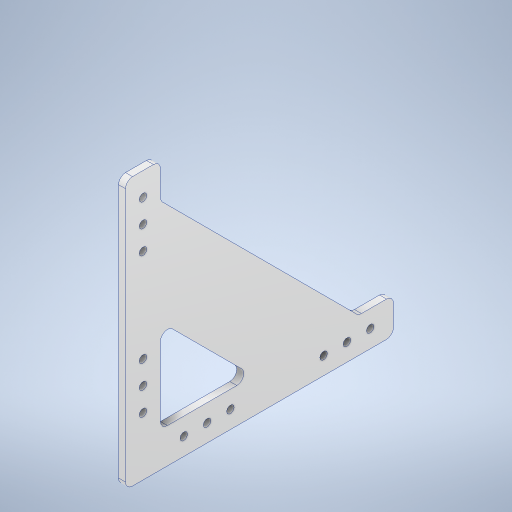
# Autodesk Inventor part: 射出_固定2
Saved by Autodesk Inventor 2023 (Build 270158000, 158)
## iProperties
Created: 2022-04-20
Part Number: 射出_固定2
Material: アルミニウム 6061
Document SubType Name: Modeling
Designer: yuta
Density: 2.7 g/cm^3
Appearance: アルミニウム - フラット
Author: yuta
Autodesk Inventor part; units mm, degrees
ref_plane "YZ Plane" through (0, 0, 0) normal (1, 0, 0) x (0, 1, 0)
ref_plane "XZ Plane" through (0, 0, 0) normal (0, 1, 0) x (-1, 0, 0)
ref_plane "XY Plane" through (0, 0, 0) normal (0, 0, 1) x (1, 0, 0)
sketch "スケッチ1" plane through (0, 0, 0) normal (1, 0, 0) x (0, 1, 0)
  line L0 (0, 0) -> (0, -115)
  line L1 (0, 0) -> (115, 0) construction
  line L2 (0, 0) -> (115, 0)
  line L3 (0, 0) -> (115, 0) construction
  line L4 (115, 0) -> (0, -115)
  dimension "d0" = 115
  dimension "d1" = 90
  dimension "d2" = 115
  dimension "d3" = 0
  constraints: 10 end point, 2 equal length, 2 horizontal, 1 collinear, 1 vertical
  measures "d0" distance of L0.start L0.end
  measures "d1" angle of L0 L1
  measures "d2" distance of L0.start L1.end
  measures "d3" distance between parallel lines of L2 L3
extrude "押し出し1" add sketch "スケッチ1" along normal blind 3
sketch "スケッチ2" plane through (3, 0, 0) normal (1, 0, 0) x (0, 0, -1)
  line L0 (0, 0) -> (0, 65)
  line L1 (0, 115) -> (0, 0) projected
  line L2 (0, 0) -> (65, 0) construction
  line L3 (0, 0) -> (65, 0)
  line L4 (0, 0) -> (115, 0) projected
  line L5 (0, 0) -> (65, 0) construction
  line L6 (65, 0) -> (0, 65)
  dimension "d6" = 65
  dimension "d7" = 90
  dimension "d8" = 65
  dimension "d9" = 0
  constraints: 10 end point, 2 collinear, 2 equal length, 2 horizontal
  measures "d6" distance of L0.start L0.end
  measures "d7" angle of L2 L0
  measures "d8" distance of L0.start L2.end
  measures "d9" distance between parallel lines of L3 L5
extrude "押し出し2" cut sketch "スケッチ2" against normal blind 3
sketch "スケッチ3" plane through (3, 0, 0) normal (1, 0, 0) x (0, 0, -1)
  line L0 (0, 115) -> (15, 115)
  line L1 (0, 115) -> (15, 115) construction
  line L2 (15, 115) -> (15, 100)
  line L3 (115, 0) -> (0, 115) projected
  line L4 (115, 0) -> (115, 15)
  line L5 (115, 0) -> (130, 0) construction
  line L6 (115, 15) -> (100, 15)
  point P0 (0, 0)
  dimension "d12" = 15
  dimension "d13" = 0
  dimension "d14" = 15
  dimension "d15" = 90
  constraints: 12 end point, 3 horizontal, 2 equal length, 2 perpendicular, 2 point on line, 1 vertical
  measures "d12" distance of L0.start L0.end
  measures "d13" distance between parallel lines of L0 L1
  measures "d14" distance of L4.start L4.end
  measures "d15" angle of L5 L4
extrude "押し出し3" add sketch "スケッチ3" against normal blind 3
sketch "スケッチ4" plane through (3, 0, 0) normal (1, 0, 0) x (0, 0, -1)
  line L0 (15, 115) -> (0, 115) projected
  line L1 (15, 100) -> (15, 115) projected
  line L2 (0, 115) -> (0, 65) projected
  line L3 (0, 0) -> (95, 95) construction
  line L4 (0, 0) -> (134.3503, 0) construction
  point P0 (7.5, 105)
  point P1 (7.5, 95)
  point P2 (7.5, 85)
  point P3 (105, 7.5)
  point P4 (95, 7.5)
  point P5 (85, 7.5)
  dimension "d18" = 10
  dimension "d19" = 7.5
  dimension "d20" = 7.5
  dimension "d21" = 7.5
  dimension "d22" = 10
  dimension "d23" = 10
  dimension "d24" = 45
  constraints: 4 end point, 3 symmetric about line, 1 equal length, 1 horizontal
  measures "d18" distance from line of L0 point (7.5, 105)
  measures "d19" distance from line of L1 point (7.5, 105)
  measures "d20" distance from line of L2 point (7.5, 95)
  measures "d21" distance from line of L2 point (7.5, 85)
  measures "d22" distance of point (7.5, 105) point (7.5, 95)
  measures "d23" distance of point (7.5, 95) point (7.5, 85)
  measures "d24" angle of L4 L3
hole "穴1" at (3, 105, -7.5) at (3, 95, -7.5) at (3, 85, -7.5) at (3, 7.5, -105) at (3, 7.5, -95) at (3, 7.5, -85) direction (-1, 0, 0) diameter 3.2 end through all
fillet "フィレット1" radius 3 8 edges at (1.5, 115, -15) (1.5, 100, -15) (1.5, 15, -100) (1.5, 15, -115) (1.5, 0, -115) (1.5, 0, -65) (1.5, 65, 0) (1.5, 115, 0)
sketch "スケッチ5" plane through (3, 0, 0) normal (1, 0, 0) x (0, 0, -1)
  line L0 (0, 0) -> (65, 0)
  line L1 (66.2426, 0) -> (112, 0) projected
  line L2 (0, 0) -> (66.2426, 0)
  arc A0 (0, 66.2426) -> (0.8787, 64.1213) centre (3, 66.2426) ccw projected
  line L3 (0, 0) -> (0, 66.2426)
  line L4 (0.8787, 64.1213) -> (64.1213, 0.8787) projected
  line L5 (0.8787, 64.1213) -> (64.1213, 0.8787)
  arc A1 (0, 66.2426) -> (0.8787, 64.1213) centre (3, 66.2426) ccw
  arc A2 (64.1213, 0.8787) -> (66.2426, 0) centre (66.2426, 3) ccw
  constraints: 8 end point, 4 point on circle, 2 centre point, 2 horizontal, 2 tangent, 1 collinear, 1 vertical
extrude "押し出し4" add sketch "スケッチ5" against normal blind 3
sketch "スケッチ6" plane through (3, 0, 0) normal (1, 0, 0) x (0, 0, -1)
  line L0 (0, 0) -> (112, 0) projected
  line L1 (0, 112) -> (0, 0) projected
  line L2 (15, 15) -> (55, 15)
  line L3 (55, 15) -> (15, 55)
  line L4 (15, 55) -> (15, 15)
  dimension "d35" = 15
  dimension "d36" = 15
  dimension "d37" = 40
  dimension "d38" = 40
  constraints: 6 end point, 1 horizontal, 1 perpendicular
  measures "d35" distance from line of L0 L2.start
  measures "d36" distance from line of L1 L2.start
  measures "d37" distance of L2.start L3.end
  measures "d38" distance of L2.start L2.end
extrude "押し出し5" cut sketch "スケッチ6" against normal blind 3
sketch "スケッチ7" plane through (3, 0, 0) normal (1, 0, 0) x (0, 0, -1)
  line L0 (0, 112) -> (0, 0) projected
  line L1 (0, 0) -> (112, 0) projected
  line L2 (0, 0) -> (0, 112) projected
  line L3 (0, 0) -> (76.3955, 76.3955) construction
  line L4 (0, 0) -> (108.0395, 0) construction
  point P0 (7.5, 25)
  point P1 (7.5, 35)
  point P2 (7.5, 45)
  point P3 (25, 7.5)
  point P4 (35, 7.5)
  point P5 (45, 7.5)
  dimension "d41" = 7.5
  dimension "d42" = 25
  dimension "d43" = 10
  dimension "d44" = 10
  dimension "d46" = 45
  constraints: 4 end point, 3 symmetric about line, 1 equal length, 1 horizontal
  measures "d41" distance from line of L0 point (7.5, 25)
  measures "d42" distance from line of L1 point (7.5, 25)
  measures "d43" distance of point (7.5, 25) point (7.5, 35)
  measures "d44" distance of point (7.5, 35) point (7.5, 45)
  measures "d46" angle of L4 L3
hole "穴2" at (3, 25, -7.5) at (3, 35, -7.5) at (3, 45, -7.5) at (3, 7.5, -25) at (3, 7.5, -35) at (3, 7.5, -45) direction (-1, 0, 0) diameter 3.2 end through all
fillet "フィレット2" radius 3 4 edges at (1.5, 15, -55) (1.5, 55, -15) (1.5, 15, -15) (1.5, 0, 0)
